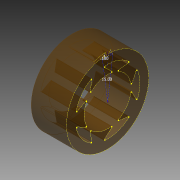
# Autodesk Inventor part: Wheel Tread test
Saved by Autodesk Inventor 2013 (Build 170138000, 138)
## iProperties
Created: 2013-04-30
Part Number: Wheel Tread test
Material: Rubber
Document SubType Name: Modeling
Designer: grtstudent
Density: 1 g/cm^3
Author: grtstudent
Autodesk Inventor part; units mm, degrees
ref_plane "YZ Plane" through (0, 0, 0) normal (1, 0, 0) x (0, 1, 0)
ref_plane "XZ Plane" through (0, 0, 0) normal (0, 1, 0) x (-1, 0, 0)
ref_plane "XY Plane" through (0, 0, 0) normal (0, 0, 1) x (1, 0, 0)
sketch "Sketch1" plane through (0, 0, 0) normal (1, 0, 0) x (0, 1, 0)
  circle A0 centre (0, 0) radius 44.45
  circle A1 centre (11.1973, -15.4118) radius 1.905
  circle A2 centre (-18.1176, 5.8868) radius 1.905
  circle A3 centre (0, 19.05) radius 1.905
  circle A4 centre (-11.1973, -15.4118) radius 1.905
  circle A5 centre (18.1176, 5.8868) radius 1.905
  line L0 (-6.4158, 0) -> (-3.2079, 5.5563)
  line L1 (-3.2079, 5.5563) -> (3.2079, 5.5563)
  line L2 (3.2079, 5.5563) -> (6.4158, 0)
  line L3 (6.4158, 0) -> (3.2079, -5.5563)
  line L4 (3.2079, -5.5563) -> (-3.2079, -5.5563)
  line L5 (-3.2079, -5.5563) -> (-6.4158, 0)
  arc A6 (-6.9808, 33.2105) -> (-7.631, 34.0811) centre (-7.5009, 33.5002) ccw
  arc A7 (-7.631, 34.0811) -> (-30.055, 17.7891) centre (0, 0) ccw
  arc A8 (-30.055, 17.7891) -> (-29.4279, 16.9018) centre (-29.5427, 17.4859) ccw
  line L6 (-18.3896, 19.0716) -> (-29.4279, 16.9018)
  arc A9 (-17.8563, 18.0641) -> (-18.3896, 19.0716) centre (-18.2748, 18.4875) ccw
  arc A10 (-17.8563, 18.0641) -> (-25.0639, -4.1185) centre (0, 0) ccw
  arc A11 (-26.0876, -4.6201) -> (-25.0639, -4.1185) centre (-25.6513, -4.215) ccw
  line L7 (-33.7423, 3.6235) -> (-26.0876, -4.6201)
  arc A12 (-33.7423, 3.6235) -> (-34.7712, 3.2742) centre (-34.1785, 3.2184) ccw
  arc A13 (-34.7712, 3.2742) -> (-26.206, -23.0869) centre (0, 0) ccw
  arc A14 (-26.206, -23.0869) -> (-25.1682, -22.7646) centre (-25.7593, -22.6933) ccw
  line L8 (-23.8209, -11.5961) -> (-25.1682, -22.7646)
  arc A15 (-22.6979, -11.4002) -> (-23.8209, -11.5961) centre (-23.2299, -11.6674) ccw
  arc A16 (-22.6979, -11.4002) -> (-3.8282, -25.1098) centre (0, 0) ccw
  arc A17 (-3.6675, -26.2384) -> (-3.8282, -25.1098) centre (-3.918, -25.6984) ccw
  line L9 (-13.873, -30.9711) -> (-3.6675, -26.2384)
  arc A18 (-13.873, -30.9711) -> (-13.8588, -32.0576) centre (-13.6226, -31.5111) ccw
  arc A19 (-13.8588, -32.0576) -> (13.8588, -32.0576) centre (0, 0) ccw
  arc A20 (13.8588, -32.0576) -> (13.873, -30.9711) centre (13.6226, -31.5111) ccw
  line L10 (3.6675, -26.2384) -> (13.873, -30.9711)
  arc A21 (3.8282, -25.1098) -> (3.6675, -26.2384) centre (3.918, -25.6984) ccw
  arc A22 (3.8282, -25.1098) -> (22.6979, -11.4002) centre (0, 0) ccw
  arc A23 (23.8209, -11.5961) -> (22.6979, -11.4002) centre (23.2299, -11.6674) ccw
  line L11 (25.1682, -22.7646) -> (23.8209, -11.5961)
  arc A24 (25.1682, -22.7646) -> (26.206, -23.0869) centre (25.7593, -22.6933) ccw
  arc A25 (26.206, -23.0869) -> (34.7712, 3.2742) centre (0, 0) ccw
  arc A26 (34.7712, 3.2742) -> (33.7423, 3.6235) centre (34.1785, 3.2184) ccw
  line L12 (26.0876, -4.6201) -> (33.7423, 3.6235)
  arc A27 (25.0639, -4.1185) -> (26.0876, -4.6201) centre (25.6513, -4.215) ccw
  arc A28 (25.0639, -4.1185) -> (17.8563, 18.0641) centre (0, 0) ccw
  arc A29 (18.3896, 19.0716) -> (17.8563, 18.0641) centre (18.2748, 18.4875) ccw
  line L13 (29.4279, 16.9018) -> (18.3896, 19.0716)
  arc A30 (29.4279, 16.9018) -> (30.055, 17.7891) centre (29.5427, 17.4859) ccw
  arc A31 (30.055, 17.7891) -> (7.631, 34.0811) centre (0, 0) ccw
  arc A32 (7.631, 34.0811) -> (6.9808, 33.2105) centre (7.5009, 33.5002) ccw
  line L14 (12.4555, 23.383) -> (6.9808, 33.2105)
  arc A33 (11.6621, 22.5645) -> (12.4555, 23.383) centre (11.9354, 23.0933) ccw
  arc A34 (11.6621, 22.5645) -> (-11.6621, 22.5645) centre (0, 0) ccw
  arc A35 (-12.4555, 23.383) -> (-11.6621, 22.5645) centre (-11.9354, 23.0933) ccw
  line L15 (-6.9808, 33.2105) -> (-12.4555, 23.383)
  dimension "d0" = 88.9
  constraints: 60 point on circle, 36 centre point, 32 end point, 1 coincident
  measures "d0" diameter of A0
extrude "Extrusion1" add sketch "Sketch1" along normal blind 38.1 contours A0
sketch "Sketch2" plane through (38.1, 0, 0) normal (1, 0, 0) x (0, 0, -1)
  line L0 (0, 0) -> (-5.8019, 44.0697) construction
  line L1 (0, 0) -> (5.8019, 44.0697) construction
  line L2 (-33.2105, -6.9808) -> (-23.383, -12.4555) construction
  arc A0 (-23.383, -12.4555) -> (-22.5645, -11.6621) centre (-23.0933, -11.9354) ccw construction
  arc A1 (-22.5645, 11.6621) -> (-22.5645, -11.6621) centre (0, 0) ccw construction
  arc A2 (-22.5645, 11.6621) -> (-23.383, 12.4555) centre (-23.0933, 11.9354) ccw construction
  line L3 (-23.383, 12.4555) -> (-33.2105, 6.9808) construction
  arc A3 (-34.0811, 7.631) -> (-33.2105, 6.9808) centre (-33.5002, 7.5009) ccw construction
  arc A4 (-17.7891, 30.055) -> (-34.0811, 7.631) centre (0, 0) ccw construction
  arc A5 (-16.9018, 29.4279) -> (-17.7891, 30.055) centre (-17.4859, 29.5427) ccw construction
  line L4 (-16.9018, 29.4279) -> (-19.0716, 18.3896) construction
  arc A6 (-19.0716, 18.3896) -> (-18.0641, 17.8563) centre (-18.4875, 18.2748) ccw construction
  arc A7 (4.1185, 25.0639) -> (-18.0641, 17.8563) centre (0, 0) ccw construction
  arc A8 (4.1185, 25.0639) -> (4.6201, 26.0876) centre (4.215, 25.6513) ccw construction
  line L5 (4.6201, 26.0876) -> (-3.6235, 33.7423) construction
  arc A9 (-3.2742, 34.7712) -> (-3.6235, 33.7423) centre (-3.2184, 34.1785) ccw construction
  arc A10 (23.0869, 26.206) -> (-3.2742, 34.7712) centre (0, 0) ccw construction
  arc A11 (22.7646, 25.1682) -> (23.0869, 26.206) centre (22.6933, 25.7593) ccw construction
  line L6 (22.7646, 25.1682) -> (11.5961, 23.8209) construction
  arc A12 (11.5961, 23.8209) -> (11.4002, 22.6979) centre (11.6674, 23.2299) ccw construction
  arc A13 (25.1098, 3.8282) -> (11.4002, 22.6979) centre (0, 0) ccw construction
  arc A14 (25.1098, 3.8282) -> (26.2384, 3.6675) centre (25.6984, 3.918) ccw construction
  line L7 (26.2384, 3.6675) -> (30.9711, 13.873) construction
  arc A15 (32.0576, 13.8588) -> (30.9711, 13.873) centre (31.5111, 13.6226) ccw construction
  arc A16 (32.0576, -13.8588) -> (32.0576, 13.8588) centre (0, 0) ccw construction
  arc A17 (30.9711, -13.873) -> (32.0576, -13.8588) centre (31.5111, -13.6226) ccw construction
  line L8 (30.9711, -13.873) -> (26.2384, -3.6675) construction
  arc A18 (26.2384, -3.6675) -> (25.1098, -3.8282) centre (25.6984, -3.918) ccw construction
  arc A19 (11.4002, -22.6979) -> (25.1098, -3.8282) centre (0, 0) ccw construction
  arc A20 (11.4002, -22.6979) -> (11.5961, -23.8209) centre (11.6674, -23.2299) ccw construction
  line L9 (11.5961, -23.8209) -> (22.7646, -25.1682) construction
  arc A21 (23.0869, -26.206) -> (22.7646, -25.1682) centre (22.6933, -25.7593) ccw construction
  arc A22 (-3.2742, -34.7712) -> (23.0869, -26.206) centre (0, 0) ccw construction
  arc A23 (-3.6235, -33.7423) -> (-3.2742, -34.7712) centre (-3.2184, -34.1785) ccw construction
  line L10 (-3.6235, -33.7423) -> (4.6201, -26.0876) construction
  arc A24 (4.6201, -26.0876) -> (4.1185, -25.0639) centre (4.215, -25.6513) ccw construction
  arc A25 (-18.0641, -17.8563) -> (4.1185, -25.0639) centre (0, 0) ccw construction
  arc A26 (-18.0641, -17.8563) -> (-19.0716, -18.3896) centre (-18.4875, -18.2748) ccw construction
  line L11 (-19.0716, -18.3896) -> (-16.9018, -29.4279) construction
  arc A27 (-17.7891, -30.055) -> (-16.9018, -29.4279) centre (-17.4859, -29.5427) ccw construction
  arc A28 (-34.0811, -7.631) -> (-17.7891, -30.055) centre (0, 0) ccw construction
  arc A29 (-33.2105, -6.9808) -> (-34.0811, -7.631) centre (-33.5002, -7.5009) ccw construction
  circle A30 centre (0, 0) radius 44.45 construction
  line L12 (0, 36.6205) -> (0, 33.3224) construction
  line L13 (-5.4704, 41.5515) -> (-2.9072, 44.3548) construction
  line L14 (-2.9072, 44.3548) -> (0, 41.91) construction
  line L15 (0, 41.91) -> (2.9072, 44.3548) construction
  line L16 (2.9072, 44.3548) -> (5.4704, 41.5515) construction
  line L17 (-5.4704, 41.5515) -> (-3.0896, 47.1379) construction
  line L18 (-3.0896, 47.1379) -> (0, 41.91) construction
  line L19 (0, 41.91) -> (3.0896, 47.1379) construction
  line L20 (3.0896, 47.1379) -> (5.4704, 41.5515) construction
  arc A31 (-1.5314, 47.2142) -> (-15.1674, 44.7379) centre (0, 0) ccw construction
  line L21 (-3.0896, 47.1379) -> (-2.7435, 41.8582) construction
  line L22 (3.0896, 47.1379) -> (2.7435, 41.8582) construction
  arc A32 (5.4704, 41.5515) -> (-5.4704, 41.5515) centre (0, 0) ccw construction
  point P0 (0, 44.45)
  dimension "d4" = 15
  dimension "d5" = 2.54
  constraints: 26 end point, 11 point on circle, 6 point on line, 2 centre point, 2 coincident, 1 vertical, 3 other
  measures "d4" angle of L1 L0
  measures "d5" radial gap between concentric circles of A30 A32
body "Solid1"
